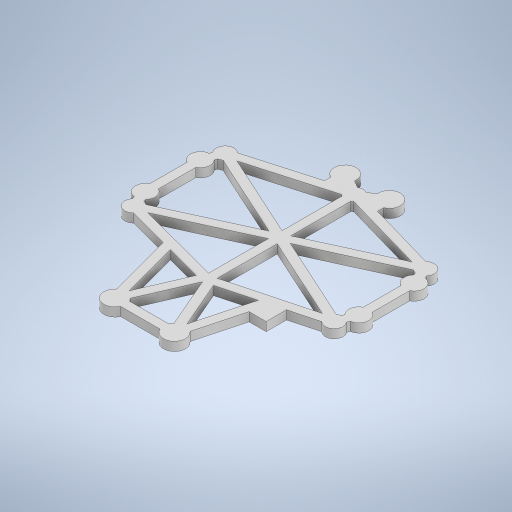
# Autodesk Inventor part: v2chassis
Saved by Autodesk Inventor 2024.2 (Build 282272000, 272)
## iProperties
Created: 2023-12-09
Part Number: v2chassis
Material: Generic
Document SubType Name: Modeling
Designer: Eric
Density: 1 g/cm^3
Appearance: Default
Author: Eric
Autodesk Inventor part; units mm, degrees
ref_plane "YZ Plane" through (0, 0, 0) normal (1, 0, 0) x (0, 1, 0)
ref_plane "XZ Plane" through (0, 0, 0) normal (0, 1, 0) x (-1, 0, 0)
ref_plane "XY Plane" through (0, 0, 0) normal (0, 0, 1) x (1, 0, 0)
sketch "Sketch1" plane through (0, 0, 0) normal (0, 1, 0) x (-1, 0, 0)
  circle A0 centre (30.4866, -33.5844) radius 1.55
  circle A1 centre (30.4866, -82.5844) radius 1.55
  circle A2 centre (-31.5134, -77.3344) radius 1.55
  circle A3 centre (-31.5134, -38.8344) radius 1.55
  circle A4 centre (30.4866, -33.5844) radius 5
  circle A5 centre (30.4866, -82.5844) radius 5
  circle A6 centre (-31.5134, -77.3344) radius 5
  circle A7 centre (-31.5134, -38.8344) radius 5
  line L0 (43, 55.7856) -> (45.4, 57.1713)
  line L1 (45.4, 57.1713) -> (47.8, 55.7856)
  line L2 (47.8, 55.7856) -> (47.8, 53.0144)
  line L3 (47.8, 53.0144) -> (45.4, 51.6287)
  line L4 (45.4, 51.6287) -> (43, 53.0144)
  line L5 (43, 53.0144) -> (43, 55.7856)
  line L6 (47.8, 14.3856) -> (47.8, 11.6144)
  line L7 (47.8, 11.6144) -> (45.4, 10.2287)
  line L8 (45.4, 10.2287) -> (43, 11.6144)
  line L9 (43, 11.6144) -> (43, 14.3856)
  line L10 (43, 14.3856) -> (45.4, 15.7713)
  line L11 (45.4, 15.7713) -> (47.8, 14.3856)
  line L12 (-43, 55.7856) -> (-43, 53.0144)
  line L13 (-43, 53.0144) -> (-45.4, 51.6287)
  line L14 (-45.4, 51.6287) -> (-47.8, 53.0144)
  line L15 (-47.8, 53.0144) -> (-47.8, 55.7856)
  line L16 (-47.8, 55.7856) -> (-45.4, 57.1713)
  line L17 (-45.4, 57.1713) -> (-43, 55.7856)
  line L18 (-1.3856, 2.4) -> (1.3856, 2.4)
  line L19 (1.3856, 2.4) -> (2.7713, 0)
  line L20 (2.7713, 0) -> (1.3856, -2.4)
  line L21 (1.3856, -2.4) -> (-1.3856, -2.4)
  line L22 (-1.3856, -2.4) -> (-2.7713, 0)
  line L23 (-2.7713, 0) -> (-1.3856, 2.4)
  line L24 (-45.4, 15.7713) -> (-43, 14.3856)
  line L25 (-43, 14.3856) -> (-43, 11.6144)
  line L26 (-43, 11.6144) -> (-45.4, 10.2287)
  line L27 (-45.4, 10.2287) -> (-47.8, 11.6144)
  line L28 (-47.8, 11.6144) -> (-47.8, 14.3856)
  line L29 (-47.8, 14.3856) -> (-45.4, 15.7713)
  circle A8 centre (45.4, 54.4) radius 4
  circle A9 centre (-45.4, 54.4) radius 4
  circle A10 centre (45.4, 13) radius 4
  circle A11 centre (-45.4, 13) radius 4
  circle A12 centre (0, 0) radius 4
  line L30 (43.0778, 16.2569) -> (4.8209, 33.7)
  line L31 (4.8209, 33.7) -> (43.0778, 51.1431)
  line L32 (41.4183, 54.7827) -> (2, 36.81)
  line L33 (2, 36.81) -> (2, 63.9359)
  line L34 (41.4183, 12.6173) -> (2, 30.59)
  line L35 (2, 30.59) -> (2, 3.4641)
  line L36 (-2, 3.4641) -> (-2, 30.59)
  line L37 (-2, 30.59) -> (-41.4183, 12.6173)
  line L38 (-43.0778, 16.2569) -> (-4.8209, 33.7)
  line L39 (-4.8209, 33.7) -> (-43.0778, 51.1431)
  line L40 (-41.4183, 54.7827) -> (-2, 36.81)
  line L41 (-2, 36.81) -> (-2, 63.9359)
  line L42 (42.6203, 10.1237) -> (3.8808, -0.9691)
  line L43 (-2.7797, 2.8763) -> (-41.5192, 13.9691)
  line L44 (-42.6203, 10.1237) -> (-3.8808, -0.9691)
  line L45 (41.5192, 13.9691) -> (2.7797, 2.8763)
  line L46 (46.7546, 43.35) -> (45.1091, 46.2)
  line L47 (45.1091, 46.2) -> (46.7546, 49.05)
  line L48 (46.7546, 49.05) -> (50.0454, 49.05)
  line L49 (50.0454, 49.05) -> (51.6909, 46.2)
  line L50 (51.6909, 46.2) -> (50.0454, 43.35)
  line L51 (50.0454, 43.35) -> (46.7546, 43.35)
  line L52 (46.7546, 24.05) -> (50.0454, 24.05)
  line L53 (50.0454, 24.05) -> (51.6909, 21.2)
  line L54 (51.6909, 21.2) -> (50.0454, 18.35)
  line L55 (50.0454, 18.35) -> (46.7546, 18.35)
  line L56 (46.7546, 18.35) -> (45.1091, 21.2)
  line L57 (45.1091, 21.2) -> (46.7546, 24.05)
  line L58 (-51.6909, 21.2) -> (-50.0454, 24.05)
  line L59 (-50.0454, 24.05) -> (-46.7546, 24.05)
  line L60 (-46.7546, 24.05) -> (-45.1091, 21.2)
  line L61 (-45.1091, 21.2) -> (-46.7546, 18.35)
  line L62 (-46.7546, 18.35) -> (-50.0454, 18.35)
  line L63 (-50.0454, 18.35) -> (-51.6909, 21.2)
  line L64 (-51.6909, 46.2) -> (-50.0454, 49.05)
  line L65 (-50.0454, 49.05) -> (-46.7546, 49.05)
  line L66 (-46.7546, 49.05) -> (-45.1091, 46.2)
  line L67 (-45.1091, 46.2) -> (-46.7546, 43.35)
  line L68 (-46.7546, 43.35) -> (-50.0454, 43.35)
  line L69 (-50.0454, 43.35) -> (-51.6909, 46.2)
  line L70 (41.5368, 53.3628) -> (2, 63.9359)
  line L71 (-2, 63.9359) -> (-41.5368, 53.3628)
  line L72 (-42.5702, 57.227) -> (-30, 60.5886)
  line L73 (-30, 60.5886) -> (-30, 69.8)
  line L74 (-30, 69.8) -> (-22.2827, 69.8)
  line L75 (-22.2827, 69.8) -> (-16.6198, 90.8927)
  line L76 (16.6198, 90.8927) -> (24.3501, 62.0995)
  line L77 (24.3501, 62.0995) -> (42.5702, 57.227)
  line L78 (-11.8546, 91.95) -> (-15.1454, 91.95)
  line L79 (-15.1454, 91.95) -> (-16.7909, 94.8)
  line L80 (-16.7909, 94.8) -> (-15.1454, 97.65)
  line L81 (-15.1454, 97.65) -> (-11.8546, 97.65)
  line L82 (-11.8546, 97.65) -> (-10.2091, 94.8)
  line L83 (-10.2091, 94.8) -> (-11.8546, 91.95)
  line L84 (16.7909, 94.8) -> (15.1454, 91.95)
  line L85 (15.1454, 91.95) -> (11.8546, 91.95)
  line L86 (11.8546, 91.95) -> (10.2091, 94.8)
  line L87 (10.2091, 94.8) -> (11.8546, 97.65)
  line L88 (11.8546, 97.65) -> (15.1454, 97.65)
  line L89 (15.1454, 97.65) -> (16.7909, 94.8)
  line L90 (19.8881, 63.2928) -> (12.7566, 89.8556)
  line L91 (-12.7566, 89.8556) -> (-19.8881, 63.2928)
  line L92 (-19.8881, 63.2928) -> (-3.9062, 67.5667)
  line L93 (-3.9062, 67.5667) -> (-13.5174, 89.8)
  line L94 (19.8881, 63.2928) -> (3.9062, 67.5667)
  line L95 (3.9062, 67.5667) -> (13.5174, 89.8)
  line L96 (0, 68.6113) -> (9.8458, 91.3872)
  line L97 (0, 68.6113) -> (-9.8458, 91.3872)
  circle A13 centre (48.4, 21.2) radius 4.5
  circle A14 centre (48.4, 46.2) radius 4.5
  circle A15 centre (-48.4, 46.2) radius 4.5
  circle A16 centre (-48.4, 21.2) radius 4.5
  line L98 (50.4, 25.2311) -> (50.4, 42.1689)
  line L99 (46.4, 25.2311) -> (46.4, 42.1689)
  line L100 (48.4684, 15.5661) -> (48.8932, 16.7271)
  line L101 (44.712, 16.9404) -> (45.1367, 18.1014)
  line L102 (48.8932, 50.6729) -> (48.4684, 51.8339)
  line L103 (45.1367, 49.2986) -> (44.712, 50.4596)
  line L104 (-48.8932, 50.6729) -> (-48.4684, 51.8339)
  line L105 (-46.4, 25.2311) -> (-46.4, 42.1689)
  line L106 (-50.4, 42.1689) -> (-50.4, 25.2311)
  line L107 (-45.1367, 18.1014) -> (-44.712, 16.9404)
  line L108 (-48.4684, 15.5661) -> (-48.8932, 16.7271)
  line L109 (-45.1367, 49.2986) -> (-44.712, 50.4596)
  circle A17 centre (13.5, 94.8) radius 5
  circle A18 centre (-13.5, 94.8) radius 5
  line L110 (8.9174, 92.8) -> (-8.9174, 92.8)
  line L111 (-8.9174, 96.8) -> (8.9174, 96.8)
  line L112 (8.3546, -8.85) -> (6.7091, -6)
  line L113 (6.7091, -6) -> (8.3546, -3.15)
  line L114 (8.3546, -3.15) -> (11.6454, -3.15)
  line L115 (11.6454, -3.15) -> (13.2909, -6)
  line L116 (13.2909, -6) -> (11.6454, -8.85)
  line L117 (11.6454, -8.85) -> (8.3546, -8.85)
  line L118 (-11.6454, -3.15) -> (-8.3546, -3.15)
  line L119 (-8.3546, -3.15) -> (-6.7091, -6)
  line L120 (-6.7091, -6) -> (-8.3546, -8.85)
  line L121 (-8.3546, -8.85) -> (-11.6454, -8.85)
  line L122 (-11.6454, -8.85) -> (-13.2909, -6)
  line L123 (-13.2909, -6) -> (-11.6454, -3.15)
  circle A19 centre (10, -6) radius 5
  circle A20 centre (-10, -6) radius 5
  line L124 (5.0415, -5.3573) -> (1.9415, -3.4973)
  line L125 (-5.0415, -5.3573) -> (-1.9415, -3.4973)
  line L126 (-12, -1.4174) -> (-12, 1.3557)
  line L127 (12, -1.4174) -> (12, 1.3557)
  point P0 (0, 92.8)
  point P1 (-39.6361, 13.4299)
  point P2 (-13.0573, 88.7356)
  point P3 (13.0573, 88.7356)
  point P4 (-39.4993, 53.9077)
  point P5 (39.6361, 13.4299)
  point P6 (39.4993, 53.9077)
  dimension "d37" = 8
  dimension "d1" = 3.1
  dimension "d2" = 49
  dimension "d3" = 62
  dimension "d5" = 5.25
  dimension "d6" = 5.25
  dimension "d7" = 10
  dimension "d13" = 13
  dimension "d14" = 90.8
  dimension "d15" = 45.4
  dimension "d17" = 4
  dimension "d18" = 4
  dimension "d19" = 4
  dimension "d20" = 2
  dimension "d21" = 2
  dimension "d22" = 2
  dimension "d23" = 2
  dimension "d24" = 2
  dimension "d25" = 4
  dimension "d26" = 2
  dimension "d27" = 2
  dimension "d30" = 4
  dimension "d31" = 2
  dimension "d32" = 2
  dimension "d35" = 5.7
  dimension "d36" = 25
  dimension "d38" = 4.8
  dimension "d39" = 69.8
  dimension "d40" = 15.4
  dimension "d41" = 4
  dimension "d42" = 4
  dimension "d43" = 2
  dimension "d44" = 2
  dimension "d48" = 30
  dimension "d49" = 27
  dimension "d51" = 3
  dimension "d52" = 3
  dimension "d53" = 4
  dimension "d55" = 4
  dimension "d56" = 4
  dimension "d57" = 4
  dimension "d65" = 8.2
  dimension "d66" = 9
  dimension "d67" = 4
  dimension "d68" = 2
  dimension "d69" = 4
  dimension "d70" = 2
  dimension "d71" = 2
  dimension "d72" = 4
  dimension "d73" = 2
  dimension "d74" = 2
  dimension "d75" = 4
  dimension "d76" = 2
  dimension "d77" = 2
  dimension "d78" = 4
  dimension "d79" = 2
  dimension "d80" = 4
  dimension "d81" = 2
  dimension "d82" = 10
  dimension "d83" = 4
  dimension "d84" = 2
  dimension "d85" = 27
  dimension "d86" = 2
  dimension "d87" = 2
  dimension "d88" = 2
  constraints: 256 end point, 56 point on circle, 22 parallel, 20 centre point, 19 coincident, 13 equal length, 11 equal radius, 11 vertical, 10 horizontal, 8 collinear, 8 vertical alignment, 6 horizontal alignment, 3 point on line, 1 midpoint, 1 perpendicular, 183 other
  measures "d1" diameter of A0
  measures "d2" distance of A0.centre A1.centre
  measures "d3" horizontal distance of A1.centre A2.centre
  measures "d5" vertical distance of A0.centre A3.centre
  measures "d6" vertical distance of A2.centre A1.centre
  measures "d7" diameter of A4
  measures "d13" vertical distance of point (0, 0) point (-45.4, 13)
  measures "d14" distance of point (-45.4, 13) point (45.4, 13)
  measures "d15" horizontal distance of point (45.4, 13) point (0, 0)
  measures "d17" distance between parallel lines of L32 L31
  measures "d18" distance between parallel lines of L34 L30
  measures "d19" distance between parallel lines of L33 L41
  measures "d20" distance from line of point (-45.4, 54.4) L39
  measures "d21" distance from line of L34 point (45.4, 13)
  measures "d22" distance from line of L31 point (45.4, 54.4)
  measures "d23" distance from line of L37 point (-45.4, 13)
  measures "d24" distance from line of L35 point (0, 0)
  measures "d25" distance between parallel lines of L42 L45
  measures "d26" distance from line of point (45.4, 13) L45
  measures "d27" distance from line of L45 point (0, 0)
  measures "d30" distance between parallel lines of L44 L43
  measures "d31" distance from line of L43 point (-45.4, 13)
  measures "d32" distance from line of L43 point (0, 0)
  measures "d35" distance between parallel lines of L48 L51
  measures "d36" distance of point (48.4, 46.2) point (48.4, 21.2)
  measures "d38" distance between parallel lines of L18 L21
  measures "d39" distance from line of point (0, 0) L74
  measures "d40" distance from line of L74 point (-45.4, 54.4)
  measures "d41" distance between parallel lines of L71 L72
  measures "d42" distance between parallel lines of L77 L70
  measures "d43" distance from line of point (45.4, 54.4) L70
  measures "d44" distance from line of point (-45.4, 54.4) L71
  measures "d48" distance from line of point (0, 0) L73
  measures "d49" distance of point (13.5, 94.8) point (-13.5, 94.8)
  measures "d51" horizontal distance of point (48.4, 46.2) point (45.4, 13)
  measures "d52" horizontal distance of point (-45.4, 13) point (-48.4, 21.2)
  measures "d53" distance between parallel lines of L95 L96
  measures "d55" distance between parallel lines of L93 L97
  measures "d56" distance between parallel lines of L76 L90
  measures "d57" distance between parallel lines of L75 L91
  measures "d65" vertical distance of point (45.4, 13) point (48.4, 21.2)
  measures "d66" diameter of A13
  measures "d67" distance between parallel lines of L99 L98
  measures "d68" distance from line of L98 point (48.4, 21.2)
  measures "d69" distance between parallel lines of L100 L101
  measures "d70" distance from line of L100 point (45.4, 13)
  measures "d71" distance from line of point (48.4, 21.2) L101
  measures "d72" distance between parallel lines of L102 L103
  measures "d73" distance from line of L102 point (48.4, 46.2)
  measures "d74" distance from line of point (45.4, 54.4) L103
  measures "d75" distance between parallel lines of L107 L108
  measures "d76" distance from line of point (-45.4, 13) L108
  measures "d77" distance from line of point (-48.4, 21.2) L107
  measures "d78" distance between parallel lines of L106 L105
  measures "d79" distance from line of L105 point (-48.4, 21.2)
  measures "d80" distance between parallel lines of L109 L104
  measures "d81" distance from line of point (-45.4, 54.4) L109
  measures "d82" diameter of A17
  measures "d83" distance between parallel lines of L111 L110
  measures "d84" distance from line of point (13.5, 94.8) L110
  measures "d85" distance between parallel lines of L74 L111
  measures "d86" distance from line of point (13.5, 94.8) L76
  measures "d87" distance from line of point (-13.5, 94.8) L75
  measures "d88" distance from line of point (-13.5, 94.8) L97
extrude "Extrusion1" add sketch "Sketch1" along normal blind 4 contours L0 L1 L2 L3 L4 L5 | L6 L7 L8 L9 L10 L11 | L12 L13 L14 L15 L16 L17 | L18 L19 L20 L21 L22 L23 | L24 L25 L26 L27 L28 L29 | A8 | A8 L32 L70 L31 L30 A10 L45 L34 L35 A12 L36 L37 L43 A11 L38 L39 A9 L71 L40 L72 L73 L74 L75 A18 L93 L91 L97 L96 A17 L90 L95 L76 L77 | L102 A14 L103 A8 | A8 L70 L32 | A14 | A17 | L95 L90 A17 | A14 L98 A13 L99 | A17 L110 A18 L111 | A10 | A13 | A18 | L101 A13 L100 A10 | A10 L34 L45 | A10 L42 A12 L45 L34 | A18 L91 L93 | A12 | L127 A19 L124 A12 L42 | A19 | A9 | A12 L44 A11 L37 L43 | L40 L71 A9 | A9 L109 A15 L104 | L125 A20 L126 L44 A12 | L37 A11 L43 | A15 | A20 | A11 | A15 L105 A16 L106 | A16 | L108 A16 L107 A11 | L46 L47 L48 L49 L50 L51 | L52 L53 L54 L55 L56 L57 | L58 L59 L60 L61 L62 L63 | L64 L65 L66 L67 L68 L69 | L78 L79 L80 L81 L82 L83 | L84 L85 L86 L87 L88 L89 | L112 L113 L114 L115 L116 L117 | L118 L119 L120 L121 L122 L123
body "Solid1"
